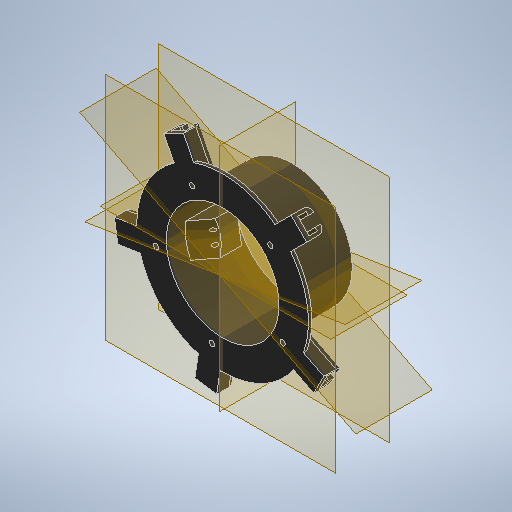
# Autodesk Inventor part: BracoRobotico_0004_001
Saved by Autodesk Inventor 2025.2 (Build 292293000, 293)
## iProperties
Created: 2025-05-28
Part Number: BracoRobotico_0004_001
Material: Rubber
Document SubType Name: Modeling
Designer: I
Density: 0.93 g/cm^3
Appearance: Rubber - Black
Author: I
Autodesk Inventor part; units mm, degrees
sketch "Sketch8" plane through (0, 0, 0) normal (0, 0, 1) x (1, 0, 0)
  circle A0 centre (0, 0) radius 70
  circle A1 centre (0, 0) radius 46
  dimension "d28" = 140
  dimension "d29" = 92
  constraints: 2 centre point, 2 coincident
  measures "d28" diameter of A0
  measures "d29" diameter of A1
extrude "Extrusion6" add sketch "Sketch8" along normal mid plane 2.75
sketch "Sketch10" plane through (0, 0, 1.375) normal (0, 0, 1) x (1, 0, 0)
  circle A0 centre (0, 0) radius 49
  circle A1 centre (0, 0) radius 46 projected
  dimension "d41" = 98
  constraints: 1 centre point, 1 coincident
  measures "d41" diameter of A0
extrude "Extrusion8" add sketch "Sketch10" against normal blind 56.75
sketch "Sketch9" plane through (0, 0, 1.375) normal (0, 0, 1) x (1, 0, 0)
  line L0 (0, 0) -> (62.2254, 62.2254) construction
  line L1 (0, 0) -> (70, 0) construction
  circle A0 centre (0, 0) radius 70 construction
  line L2 (40.4227, 27.6948) -> (68.5894, 55.8614)
  line L3 (68.5894, 55.8614) -> (55.8614, 68.5894)
  line L4 (55.8614, 68.5894) -> (27.6948, 40.4227)
  line L5 (27.6948, 40.4227) -> (40.4227, 27.6948)
  line L6 (40.4227, 27.6948) -> (55.8614, 68.5894) construction
  line L7 (68.5894, 55.8614) -> (27.6948, 40.4227) construction
  circle A1 centre (0, 0) radius 49 projected
  circle A2 centre (38.8909, 38.8909) radius 2.15
  line L8 (0, 0) -> (38.8909, 38.8909) construction
  point P0 (48.1421, 48.1421)
  point P1 (42.7227, 55.4506)
  point P2 (55.4506, 42.7227)
  dimension "d32" = 45
  dimension "d33" = 88
  dimension "d34" = 18
  dimension "d51" = 55
  dimension "d52" = 4.3
  constraints: 18 end point, 3 midpoint, 3 perpendicular, 2 coincident, 1 centre point, 1 collinear, 1 horizontal, 1 point on line, 4 other
  measures "d32" angle of L1 L0
  measures "d33" distance of L0.end L0.start
  measures "d34" distance of L2.end L3.end
  measures "d51" distance of L0.start L8.end
  measures "d52" diameter of A2
extrude "Extrusion7" add sketch "Sketch9" against normal blind 3.75 contours A1 L4 L3 L2 | L5 A1 | A2 picked at (34.9441, 33.5227)
sketch "Sketch11" plane through (68.5894, 55.8614, -2.375) normal (0.7071068, 0.7071068, 0) x (-0.7071068, 0.7071068, 0)
  line L0 (18, 3.75) -> (18, -11.25)
  line L1 (18, -11.25) -> (13, -11.25)
  line L2 (13, -11.25) -> (13, -6.75)
  line L3 (13, -6.75) -> (15.5, -6.75)
  line L4 (15.5, -6.75) -> (15.5, 0)
  line L5 (18, 0) -> (0, 0) construction
  line L6 (15.5, 0) -> (9, 0)
  line L7 (9, 0) -> (9, 3.75)
  line L8 (9, 3.75) -> (18, 3.75)
  line L9 (0, 3.75) -> (18, 3.75) projected
  point P0 (9, 2.375)
  point P1 (9, 0)
  point P2 (9, 3.75)
  dimension "d44" = 15
  dimension "d45" = 5
  dimension "d46" = 4.5
  dimension "d47" = 2.5
  constraints: 16 end point, 4 midpoint, 3 vertical, 2 horizontal, 1 coincident, 1 collinear, 1 perpendicular, 1 point on line
  measures "d44" distance of L0.start L0.end
  measures "d45" distance of L0.end L1.end
  measures "d46" distance of L1.end L2.end
  measures "d47" distance between parallel lines of L0 L4
extrude "Extrusion9" add sketch "Sketch11" against normal up to surface round surface about axis through (0, 0, 1.375) along (0, 0, -1) radius 49 far side no
ref_plane "Work Plane1" through (49.0867, 49.0867, -1.375) normal (-0.7071068, 0.7071068, 0) x (-0.7071068, -0.7071068, 0)
mirror "Mirror1" about plane through (49.0867, 49.0867, -1.375) normal (-0.7071068, 0.7071068, 0) of "Extrusion9"
sketch "Sketch12" plane through (57.6292, 66.8216, -9.125) normal (0.7071068, 0.7071068, 0) x (-0.7071068, 0.7071068, 0)
  line L0 (0, 6.75) -> (-13, 6.75) projected
  line L1 (0, 6.75) -> (0, 0) projected
  line L2 (0, 0) -> (-2.5, 0) projected
  line L3 (-2.5, 0) -> (-2.5, -4.5) projected
  line L4 (-2.5, -4.5) -> (2.5, -4.5) projected
  line L5 (2.5, 10.5) -> (2.5, -4.5) projected
  line L6 (-15.5, 10.5) -> (2.5, 10.5) projected
  line L7 (-15.5, 10.5) -> (-15.5, -4.5) projected
  line L8 (-10.5, -4.5) -> (-15.5, -4.5) projected
  line L9 (-10.5, 0) -> (-10.5, -4.5) projected
  line L10 (-13, 0) -> (-10.5, 0) projected
  line L11 (-13, 6.75) -> (-13, 0) projected
  point P0 (-6.5, 9.125)
extrude "Extrusion11" cut sketch "Sketch12" against normal blind 0.05
extrude "Extrusion10" cut sketch "Sketch9" along normal through all both and the other way through all contours A2
fillet "Fillet5" radius 5 2 edges at (41.7597, 54.4877, -13.625) (54.4877, 41.7597, -13.625)
pattern_circular "Circular Pattern1" count 5 over 360 about axis through (0, 0, -10) along (0, 0, 1) of "Extrusion7", "Extrusion9", "Mirror1", "Extrusion10", "Fillet5"
ref_plane "Work Plane2" through (78.4086, -39.9512, 1.375) normal (0.4539905, 0.8910065, 0) x (0.8910065, -0.4539905, 0)
ref_plane "Work Plane3" through (0, 0, -43.375) normal (0, 0, 1) x (1, 0, 0)
ref_plane "Work Plane4" through (-86.9166, -13.7662, 1.375) normal (-0.1564345, 0.9876883, 0) x (0.9876883, 0.1564345, 0)
sketch "Sketch13" plane through (0, 0, -43.375) normal (0, 0, 1) x (1, 0, 0)
  circle A0 centre (0, 0) radius 46 projected
  line L0 (-45.6152, 5.9373) -> (-33.3928, 7.8732)
  line L1 (-33.3928, 7.8732) -> (-29.3255, -17.8067)
  line L2 (-29.3255, -17.8067) -> (-41.5479, -19.7426)
  line L3 (-138.4163, -21.923) -> (131.8281, 20.8795) construction
  circle A1 centre (-33.0462, -10.2963) radius 1.5
  circle A2 centre (-34.6105, -0.4194) radius 1.5
  line L4 (-34.6105, -0.4194) -> (-33.0462, -10.2963) construction
  point P0 (-31.3591, -4.9668)
  point P1 (-33.8283, -5.3579)
  dimension "d60" = 26
  dimension "d61" = 31.75
  dimension "d67" = 3
  dimension "d68" = 10
  dimension "d69" = 2.5
  constraints: 8 end point, 3 perpendicular, 2 centre point, 2 coincident, 2 midpoint, 2 point on circle, 2 point on line, 1 equal radius, 1 parallel
  measures "d60" distance of L0.end L1.end
  measures "d61" distance from line of point (0, 0) L1
  measures "d67" diameter of A1
  measures "d68" distance of L4.start L4.end
  measures "d69" distance between parallel lines of L1 L4
extrude "Extrusion12" add sketch "Sketch13" along normal blind 29.25 contours L0 L1 L2 A0 picked at (-41.6092, -7.9752)
sketch "Sketch14" plane through (-31.3591, -4.9668, -43.375) normal (0.1564345, -0.9876883, 0) x (0.9876883, 0.1564345, 0)
  line L0 (0, 15) -> (-14.25, 29.25)
  line L1 (0, 0) -> (0, 29.25) construction
  line L2 (-14.25, 29.25) -> (-12.3748, 29.25) construction
  line L3 (-14.25, 29.25) -> (0, 29.25)
  line L4 (0, 29.25) -> (0, 15)
  line L5 (31.75, -23.35) -> (31.75, 56.1) projected
  point P0 (31.75, 43.375)
  dimension "d64" = 15
  constraints: 6 end point, 1 point on line
  measures "d64" distance of L1.start L0.start
revolve "Revolution1" cut sketch "Sketch14" angle 45 mid plane about axis through (0, 0, -10) along (0, 0, 1)
sketch "Sketch15" plane through (0, 0, -43.375) normal (0, 0, 1) x (1, 0, 0)
  line L0 (-138.4163, -21.923) -> (131.8281, 20.8795) construction
  line L1 (44.1069, 13.0606) -> (18.0744, 8.9375)
  line L2 (18.0744, 8.9375) -> (16.9794, 15.8513)
  line L3 (16.9794, 15.8513) -> (9.0778, 14.5998)
  line L4 (9.0778, 14.5998) -> (11.1115, 1.7599)
  circle A0 centre (0, 0) radius 46 construction
  arc A1 (45.9841, 1.2084) -> (44.1069, 13.0606) centre (0, 0) ccw
  line L5 (11.1115, 1.7599) -> (45.4337, 7.196)
  circle A2 centre (12.7985, 7.0894) radius 1.5
  line L6 (12.7985, 7.0894) -> (13.5807, 2.151) construction
  point P0 (45.4337, 7.196)
  dimension "d72" = 13
  dimension "d75" = 6
  dimension "d77" = 5
  dimension "d78" = 11.25
  dimension "d79" = 8
  dimension "d80" = 2.5
  dimension "d81" = 3
  constraints: 12 end point, 7 point on circle, 4 perpendicular, 3 point on line, 2 centre point, 1 coincident, 1 collinear, 1 parallel
  measures "d72" distance of L3.end L4.end
  measures "d75" distance between parallel lines of L0 L1
  measures "d77" distance of L6.start L6.end
  measures "d78" distance of point (0, 0) L4.end
  measures "d79" distance of L2.end L3.end
  measures "d80" distance between parallel lines of L4 L6
  measures "d81" diameter of A2
extrude "Extrusion14" add sketch "Sketch15" along normal blind 14
mirror "Mirror2" about plane through (11.1115, 1.7599, -43.375) normal (0.1564345, -0.9876883, 0) of "Extrusion14"
fillet "Fillet6" radius 7 2 edges at (19.9516, -2.9148, -36.375) (18.0744, 8.9375, -36.375)
chamfer "Chamfer1" distance 15 angle 45 1 edges at (45.4337, 7.196, -29.375)
fillet "Fillet7" radius 10 1 edges at (30.6183, 4.8495, -29.375)
body "Solid2"
